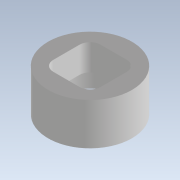
# Autodesk Inventor part: ServoArm
Saved by Autodesk Inventor 2020 (Build 240168000, 168)
## iProperties
Created: 2019-12-15
Part Number: ServoArm
Material: Generic
Document SubType Name: Modeling
Designer: Kjell
Density: 1 g/cm^3
Appearance: Default
Author: Kjell
Autodesk Inventor part; units mm, degrees
ref_plane "YZ Plane" through (0, 0, 0) normal (1, 0, 0) x (0, 1, 0)
ref_plane "XZ Plane" through (0, 0, 0) normal (0, 1, 0) x (-1, 0, 0)
ref_plane "XY Plane" through (0, 0, 0) normal (0, 0, 1) x (1, 0, 0)
ref_plane "Work Plane1" through (0, 0, 0) normal (0, 0, 1) x (1, 0, 0)
sketch "Sketch1" plane through (0, 0, 0) normal (0, 0, 1) x (1, 0, 0)
  arc A0 (-2.5, 4.5) -> (-4.5, 2.5) centre (-2.5, 2.5) ccw projected
  arc A1 (-2.5, 4.5) -> (-4.5, 2.5) centre (-2.5, 2.5) ccw projected
  line L0 (-2.5, 4.5) -> (2.5, 4.5) projected
  arc A2 (4.5, 2.5) -> (2.5, 4.5) centre (2.5, 2.5) ccw projected
  line L1 (4.5, 2.5) -> (4.5, -2.5) projected
  arc A3 (2.5, -4.5) -> (4.5, -2.5) centre (2.5, -2.5) ccw projected
  line L2 (2.5, -4.5) -> (-2.5, -4.5) projected
  arc A4 (-4.5, -2.5) -> (-2.5, -4.5) centre (-2.5, -2.5) ccw projected
  line L3 (-4.5, -2.5) -> (-4.5, 2.5) projected
  circle A5 centre (0, 0) radius 5.675 projected
  circle A6 centre (0, 0) radius 8
  circle A7 centre (0, 0) radius 6
  line L4 (-4.55, 2.5) -> (-4.55, -2.5)
  arc A8 (-4.55, -2.5) -> (-2.5, -4.55) centre (-2.5, -2.5) ccw
  line L5 (-2.5, -4.55) -> (2.5, -4.55)
  arc A9 (2.5, -4.55) -> (4.55, -2.5) centre (2.5, -2.5) ccw
  line L6 (4.55, -2.5) -> (4.55, 2.5)
  arc A10 (4.55, 2.5) -> (2.5, 4.55) centre (2.5, 2.5) ccw
  line L7 (2.5, 4.55) -> (-2.5, 4.55)
  point P0 (0, 0)
  dimension "d0" = 16
  dimension "d1" = 12
  dimension "d2" = 0.05
  constraints: 8 end point, 6 point on circle, 5 centre point, 2 coincident, 6 other
  measures "d0" diameter of A6
  measures "d1" diameter of A7
  measures "d2" distance between parallel lines of L2 L5
extrude "Extrusion1" add sketch "Sketch1" against normal blind 5 contours A5 | A6 | A7
sketch "Sketch2" plane through (0, 0, -5) normal (0, 0, -1) x (-1, 0, 0)
  circle A0 centre (0, 0) radius 8 projected
  circle A1 centre (0, 0) radius 6
  dimension "d5" = 12
  constraints: 1 centre point, 1 coincident
  measures "d5" diameter of A1
extrude "Extrusion2" add sketch "Sketch2" along normal blind 3
body "Solid1"
